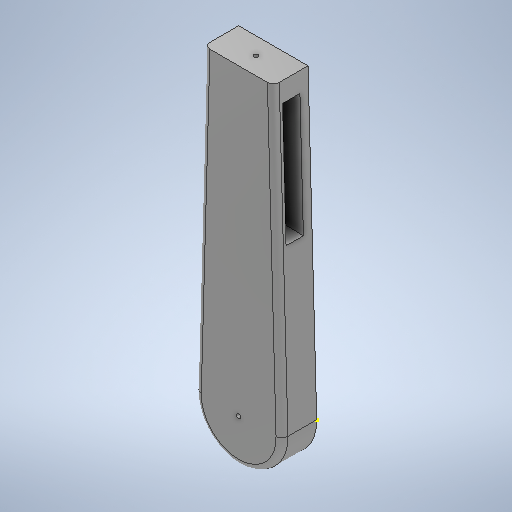
# Autodesk Inventor part: Robot_arm_2
Saved by Autodesk Inventor 2025 (Build 290162010, 162A)
## iProperties
Created: 2024-07-13
Part Number: Robot_arm_2
Material: Generic
Document SubType Name: Modeling
Designer: saees
Density: 1 g/cm^3
Appearance: Anodized - Light Gray
Author: saees
Autodesk Inventor part; units mm, degrees
ref_plane "YZ Plane" through (0, 0, 0) normal (1, 0, 0) x (0, 1, 0)
ref_plane "XZ Plane" through (0, 0, 0) normal (0, 1, 0) x (-1, 0, 0)
sketch "Sketch1" plane through (0, 0, 0) normal (0, 0, 1) x (1, 0, 0)
  arc A0 (-49.9795, 1.4309) -> (49.9795, 1.4309) centre (0, 0) ccw
  line L0 (-49.9795, 1.4309) -> (-40, 350)
  line L1 (-40, 350) -> (40, 350)
  line L2 (40, 350) -> (49.9795, 1.4309)
  point P0 (0, 350)
  dimension "d0" = 100
  dimension "d1" = 350
  dimension "d2" = 80
  constraints: 6 end point, 2 point on circle, 2 tangent, 1 centre point, 1 coincident, 1 horizontal, 1 midpoint, 1 vertical alignment
  measures "d0" diameter of A0
  measures "d1" distance of point (0, 350) point (0, 0)
  measures "d2" distance of L0.end L1.end
extrude "Extrusion1" add sketch "Sketch1" along normal blind 40
sketch "Sketch2" plane through (0, 0, 0) normal (0, 0, -1) x (-1, 0, 0)
  circle A0 centre (0, 0) radius 40
  dimension "d5" = 80
  constraints: 1 centre point, 1 coincident
  measures "d5" diameter of A0
extrude "Extrusion2" cut sketch "Sketch2" against normal blind 20
sketch "Sketch3" plane through (0, 0, 20) normal (0, 0, -1) x (-1, 0, 0)
  circle A0 centre (0, 0) radius 2.5
  dimension "d8" = 5
  constraints: 1 centre point, 1 coincident
  measures "d8" diameter of A0
extrude "Extrusion3" cut sketch "Sketch3" against normal blind 20
sketch "Sketch4" plane through (40, 350, 40) normal (0.9996, 0.0286, 0) x (0, 0, -1)
  point P0 (40, -348.7119)
ref_plane "Work Plane1" through (-49.9795, 1.4309, 0) normal (-0.9996, 0.0286, 0) x (-0.0286, -0.9996, 0)
sketch "Sketch5" plane through (-49.9795, 1.4309, 0) normal (-0.9996, 0.0286, 0) x (-0.0286, -0.9996, 0)
  point P0 (0, 0)
sketch "Sketch6" plane through (-49.9795, 1.4309, 0) normal (-0.9996, 0.0286, 0) x (-0.0286, -0.9996, 0)
  line L0 (0, -8) -> (0, 48) projected
  line L1 (-348.7119, 40) -> (0, 40) projected
  line L2 (-348.7119, 0) -> (0, 0) projected
  line L3 (-188.7119, 30) -> (-328.7119, 30)
  line L4 (-328.7119, 30) -> (-328.7119, 10)
  line L5 (-328.7119, 10) -> (-188.7119, 10)
  line L6 (-188.7119, 10) -> (-188.7119, 30)
  line L7 (-348.7119, 0) -> (-348.7119, 40) projected
  point P0 (-348.7119, 20)
  point P1 (-328.7119, 20)
  dimension "d12" = 20
  dimension "d13" = 20
  dimension "d14" = 140
  dimension "d15" = 20
  constraints: 8 end point, 2 midpoint, 2 parallel, 1 horizontal, 1 perpendicular
  measures "d12" distance from line of point (-328.712, 20) L7
  measures "d13" distance of L5.end L3.start
  measures "d14" distance of L3.start L3.end
  measures "d15" distance from line of L1 point (-328.712, 20)
extrude "Extrusion4" cut sketch "Sketch6" against normal through all contours L6 L5 L4 L3
sketch "Sketch7" plane through (-40, 350, 0) normal (0, 1, 0) x (1, 0, 0)
  line L0 (0, -20) -> (80, -20) projected
  circle A0 centre (40, -20) radius 2.5
  point P0 (40, 0)
  dimension "d18" = 5
  constraints: 1 centre point, 1 midpoint
  measures "d18" diameter of A0
extrude "Extrusion5" cut sketch "Sketch7" against normal blind 30
fillet "Fillet1" radius 6.858 3 edges at (0, -50, 40) (44.9898, 175.7155, 40) (-44.9898, 175.7155, 40)
body "Solid1"
